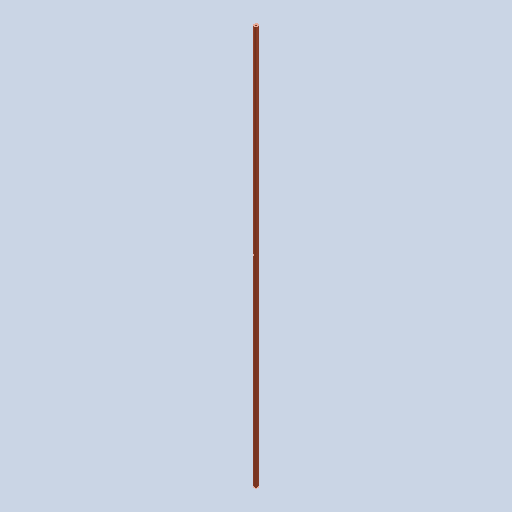
# Autodesk Inventor part: TorsOsc-2025-Rod
Saved by Autodesk Inventor 2026 (Build 300175050, 175E)
## iProperties
Created: 2023-08-18
Part Number: TorsOsc-2025-Rod
Material: Copper, Alloy
Document SubType Name: Modeling
Designer: schanen
Density: 8.92 g/cm^3
Appearance: Copper - Satin
Author: schanen
Autodesk Inventor part; units mm, degrees
ref_plane "YZ Plane" through (0, 0, 0) normal (1, 0, 0) x (0, 1, 0)
ref_plane "XZ Plane" through (0, 0, 0) normal (0, 1, 0) x (-1, 0, 0)
ref_plane "XY Plane" through (0, 0, 0) normal (0, 0, 1) x (1, 0, 0)
sketch "Sketch1" plane through (0, 0, 0) normal (0, 0, 1) x (1, 0, 0)
  line L0 (-0.425, 0) -> (-0.625, 0)
  line L1 (-0.625, 0) -> (-0.625, 132)
  line L2 (-0.625, 132) -> (-0.425, 132)
  line L3 (-0.425, 132) -> (-0.425, 0)
  line L4 (0, -26.4) -> (0, 158.4) projected
  point P0 (0, 0)
  dimension "d1" = 0.625
  dimension "d2" = 0.2
  dimension "d3" = 132
  constraints: 8 end point, 2 parallel, 1 horizontal, 1 horizontal alignment, 1 perpendicular
  measures "d1" distance from line of point (0, 0) L1
  measures "d2" distance between parallel lines of L1 L3
  measures "d3" distance of L0.end L1.end
revolve "Revolution1" add sketch "Sketch1" angle 360 about axis through (0, -10, 0) along (0, 1, 0)
sketch "Sketch2" plane through (0, 0, 0) normal (1, 0, 0) x (0, 1, 0)
  point P0 (0, 0)
  point P1 (66, 0)
  dimension "d5" = 66
  constraints: 1 horizontal alignment
  measures "d5" distance of point (0, 0) point (66, 0)
hole "Hole1" at (0, 66, 0) direction (-1, 0, 0) diameter 0.5 end through all
equation "\"d5\" = 0.5 * d3"
body "Solid1"
